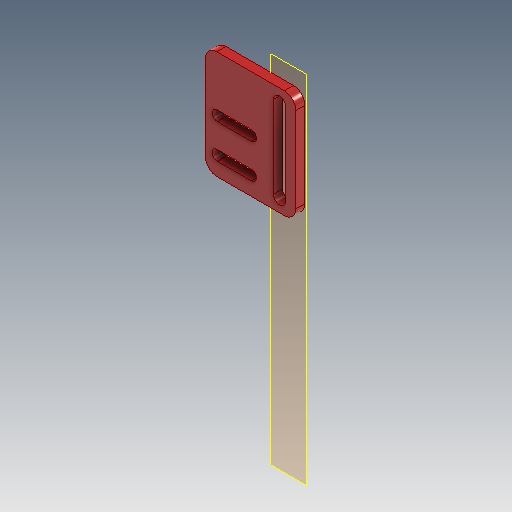
# Autodesk Inventor part: Limit switch mount top front
Saved by Autodesk Inventor 2020 (Build 240168000, 168)
## iProperties
Created: 2019-11-21
Part Number: Limit switch mount top front
Material: Generic
Document SubType Name: Modeling
Designer: ball
Density: 1 g/cm^3
Appearance: Default
Author: ball
Autodesk Inventor part; units mm, degrees
ref_plane "YZ Plane" through (0, 0, 0) normal (1, 0, 0) x (0, 1, 0)
ref_plane "XZ Plane" through (0, 0, 0) normal (0, 1, 0) x (-1, 0, 0)
ref_plane "XY Plane" through (0, 0, 0) normal (0, 0, 1) x (1, 0, 0)
ref_plane "Work Plane1" through (0, 0, 0) normal (0, 0, 1) x (1, 0, 0)
sketch "Sketch1" plane through (0, 0, 0) normal (0, 0, 1) x (1, 0, 0)
  circle A0 centre (-4.5, 66.95) radius 1.4605 construction
  circle A1 centre (-4.5, 79.65) radius 1.4605 construction
  circle A2 centre (-17.8816, 65.1334) radius 1.1938 construction
  circle A3 centre (-17.8816, 74.6584) radius 1.1938 construction
  line L0 (0, 90) -> (0, 0) construction
  line L1 (0, 90) -> (-9, 90) construction
  line L2 (-25.1016, 59.9518) -> (-15.4496, 59.9518) construction
  line L3 (-25, 90) -> (-25, -80) construction
  line L4 (-25.1016, 59.9518) -> (0, 59.9518)
  line L5 (0, 59.9518) -> (0, 90)
  line L6 (0, 90) -> (-25.1016, 90)
  line L7 (-25.1016, 90) -> (-25.1016, 59.9518)
  circle A4 centre (-4.5, 86.395) radius 1.7 construction
  circle A5 centre (-4.5, 63.5568) radius 1.7 construction
  line L8 (-4.5, 63.5568) -> (-4.5, 86.395) construction
  line L9 (-2.8, 63.5568) -> (-2.8, 86.395)
  line L10 (-6.2, 86.395) -> (-6.2, 63.5568)
  arc A6 (-6.2, 63.5568) -> (-2.8, 63.5568) centre (-4.5, 63.5568) ccw
  arc A7 (-2.8, 86.395) -> (-6.2, 86.395) centre (-4.5, 86.395) ccw
  circle A8 centre (-21.7869, 65.1334) radius 1.4097 construction
  circle A9 centre (-12.3147, 65.1334) radius 1.4097 construction
  line L11 (-9, 0) -> (-9, 90) construction
  line L12 (-12.3147, 65.1334) -> (-21.7869, 65.1334) construction
  line L13 (-12.3147, 66.5431) -> (-21.7869, 66.5431)
  line L14 (-21.7869, 63.7237) -> (-12.3147, 63.7237)
  arc A10 (-12.3147, 63.7237) -> (-12.3147, 66.5431) centre (-12.3147, 65.1334) ccw
  arc A11 (-21.7869, 66.5431) -> (-21.7869, 63.7237) centre (-21.7869, 65.1334) ccw
  line L15 (-12.3147, 76.0681) -> (-21.7869, 76.0681)
  line L16 (-21.7869, 73.2487) -> (-12.3147, 73.2487)
  arc A12 (-12.3147, 73.2487) -> (-12.3147, 76.0681) centre (-12.3147, 74.6584) ccw
  arc A13 (-21.7869, 76.0681) -> (-21.7869, 73.2487) centre (-21.7869, 74.6584) ccw
  point P0 (-4.5, 74.9759)
  point P1 (-17.0508, 65.1334)
  dimension "d0" = 3.4
  dimension "d1" = 3.4
  dimension "d2" = 3.605
  dimension "d3" = 3.605
  dimension "d4" = 3.4
  dimension "d7" = 2.8194
  dimension "d8" = 2.8194
  dimension "d9" = 3.3147
  dimension "d10" = 5.1816
  dimension "d11" = 5.1816
  dimension "d12" = 5.1816
  dimension "d13" = 3.3147
  dimension "d14" = 2.8194
  dimension "d15" = 2.8194
  constraints: 30 end point, 12 point on circle, 12 tangent, 10 centre point, 5 parallel, 2 concentric, 2 horizontal, 2 midpoint, 2 vertical, 1 perpendicular, 2 other
  measures "d0" diameter of A4
  measures "d1" diameter of A5
  measures "d2" distance from line of L8.end L1
  measures "d3" distance from line of L4 L8.start
  measures "d4" diameter of A7
  measures "d7" diameter of A8
  measures "d8" diameter of A9
  measures "d9" distance from line of L7 L12.end
  measures "d10" distance from line of L4 A2.centre
  measures "d11" distance from line of L2 L12.end
  measures "d12" distance from line of L4 L12.start
  measures "d13" distance from line of L11 L12.start
  measures "d14" diameter of A11
  measures "d15" diameter of A13
ref_plane "Work Plane2" through (-19.6152, 72.9248, 2.54) normal (0, 0, -1) x (0, 1, 0)
ref_plane "Work Plane3" through (-19.6152, 72.9248, 2.54) normal (0, 0, -1) x (0, 1, 0)
extrude "Extrusion2" add sketch "Sketch1" along normal up to surface (2.54 mm away)
fillet "Fillet1" radius 3.175 4 edges at (-25.1016, 90, 1.27) (-25.1016, 59.9518, 1.27) (0, 59.9518, 1.27) (0, 90, 1.27)
equation "\"d3\" = d2"
equation "\"d11\" = d10"
equation "\"d12\" = d10"
equation "\"d13\" = d9"
body "Solid2"
